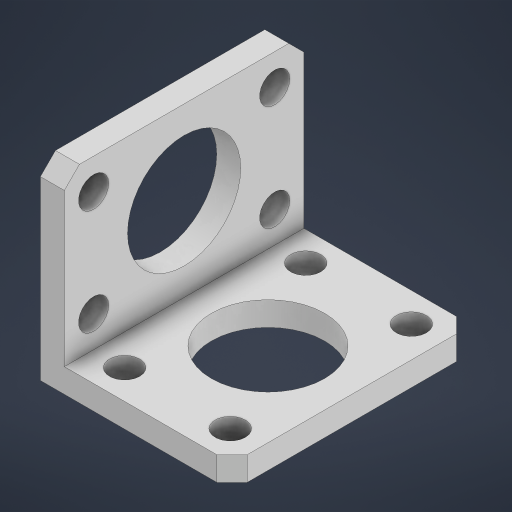
# Autodesk Inventor part: Custom L Bracket
Saved by Autodesk Inventor 2024 (Build 280153000, 153)
## iProperties
Created: 2023-09-26
Part Number: Custom L Bracket
Material: Generic
Document SubType Name: Modeling
Designer: avsar
Density: 1 g/cm^3
Appearance: Default
Author: avsar
Autodesk Inventor part; units mm, degrees
ref_plane "YZ Plane" through (0, 0, 0) normal (1, 0, 0) x (0, 1, 0)
ref_plane "XZ Plane" through (0, 0, 0) normal (0, 1, 0) x (-1, 0, 0)
ref_plane "XY Plane" through (0, 0, 0) normal (0, 0, 1) x (1, 0, 0)
sketch "Sketch1" plane through (0, 0, 0) normal (0, 1, 0) x (-1, 0, 0)
  line L0 (-12.7, 15.875) -> (12.7, 15.875)
  line L1 (12.7, 15.875) -> (12.7, -15.875)
  line L2 (12.7, -15.875) -> (-12.7, -15.875)
  line L3 (-12.7, -15.875) -> (-12.7, 15.875)
  line L4 (-12.7, 15.875) -> (12.7, -15.875) construction
  line L5 (12.7, 15.875) -> (-12.7, -15.875) construction
  point P0 (0, 0)
  dimension "d0" = 25.4
  dimension "d1" = 31.75
  constraints: 12 end point, 2 midpoint, 2 parallel, 1 horizontal, 1 perpendicular
  measures "d0" distance of L1.end L2.end
  measures "d1" distance of L0.end L1.end
extrude "Extrusion1" add sketch "Sketch1" along normal mid plane 3.175
sketch "Sketch2" plane through (0, 1.5875, 0) normal (0, 1, 0) x (1, 0, 0)
  line L0 (-12.7, 15.875) -> (-12.7, -15.875) projected
  line L1 (-12.7, -15.875) -> (-9.525, -15.875)
  line L2 (-9.525, -15.875) -> (-9.525, 15.875)
  line L3 (-9.525, 15.875) -> (-12.7, 15.875)
  line L4 (-12.7, 15.875) -> (-12.7, -15.875)
  line L5 (12.7, 15.875) -> (-12.7, 15.875) projected
  point P0 (0, 0)
  point P1 (-12.7, 15.875)
  dimension "d4" = 3.175
  constraints: 8 end point, 2 parallel, 1 horizontal, 1 perpendicular, 1 point on line
  measures "d4" distance of L3.end L2.end
extrude "Extrusion2" add sketch "Sketch2" along normal blind 22.225
sketch "Sketch3" plane through (0, 1.5875, 0) normal (0, 1, 0) x (1, 0, 0)
  line L0 (-9.525, -15.875) -> (12.7, -15.875) construction
  line L1 (12.7, 15.875) -> (-9.525, 15.875) construction
  line L2 (-9.525, 15.875) -> (-9.525, -15.875) construction
  line L3 (-9.525, -15.875) -> (12.7, -15.875) projected
  line L4 (12.7, -15.875) -> (12.7, 15.875) construction
  line L5 (12.7, 15.875) -> (-9.525, 15.875) projected
  line L6 (1.5875, 15.875) -> (1.5875, -15.875) construction
  line L7 (12.7, -15.875) -> (-12.7, -15.875) projected
  line L8 (12.7, 0) -> (-9.525, 0) construction
  circle A0 centre (1.5875, 0) radius 7.5
  circle A1 centre (-5.4125, -12) radius 2
  circle A2 centre (-5.4125, 12) radius 2
  circle A3 centre (8.5875, -12) radius 2
  circle A4 centre (8.5875, 12) radius 2
  circle A5 centre (1.5875, 0) radius 8.5 construction
  circle A6 centre (-5.4125, -12) radius 3.5 construction
  point P0 (0, 0)
  dimension "d8" = 15
  dimension "d11" = 4
  dimension "d12" = 7
  dimension "d13" = 12
  dimension "d16" = 17
  dimension "d17" = 7
  constraints: 7 centre point, 5 midpoint, 4 end point, 3 symmetric about line, 2 coincident, 1 perpendicular, 1 point on line, 3 other
  measures "d8" diameter of A0
  measures "d11" diameter of A1
  measures "d12" horizontal distance of A0.centre A1.centre
  measures "d13" vertical distance of A0.centre A1.centre
  measures "d16" diameter of A5
  measures "d17" diameter of A6
extrude "Extrusion3" cut sketch "Sketch3" against normal up to surface (3.175 mm away)
sketch "Sketch4" plane through (-9.525, 1.5875, 15.875) normal (1, 0, 0) x (0, 0, -1)
  line L0 (31.75, 0) -> (0, 0) construction
  line L1 (31.75, 0) -> (31.75, 22.225) construction
  line L2 (0, 22.225) -> (31.75, 22.225) construction
  line L3 (0, 0) -> (0, 22.225) construction
  line L4 (0, 11.1125) -> (31.75, 11.1125) construction
  line L5 (15.875, 22.225) -> (15.875, 0) construction
  circle A0 centre (15.875, 11.1125) radius 7.5
  circle A1 centre (3.875, 18.1125) radius 2
  circle A2 centre (3.875, 4.1125) radius 2
  circle A3 centre (27.875, 18.1125) radius 2
  circle A4 centre (27.875, 4.1125) radius 2
  point P0 (15.875, -1.5875)
  dimension "d18" = 15
  dimension "d19" = 4
  dimension "d20" = 12
  dimension "d21" = 7
  constraints: 6 midpoint, 5 centre point, 4 end point, 3 symmetric about line, 3 other
  measures "d18" diameter of A0
  measures "d19" diameter of A1
  measures "d20" horizontal distance of point (15.875, 11.113) A1.centre
  measures "d21" vertical distance of A0.centre A1.centre
extrude "Extrusion4" cut sketch "Sketch4" against normal up to surface (3.175 mm away)
chamfer "Chamfer1" distance 2 angle 45 4 edges at (12.7, 0, 15.875) (12.7, 0, -15.875) (-11.1125, 23.8125, -15.875) (-11.1125, 23.8125, 15.875)
body "Solid1"
